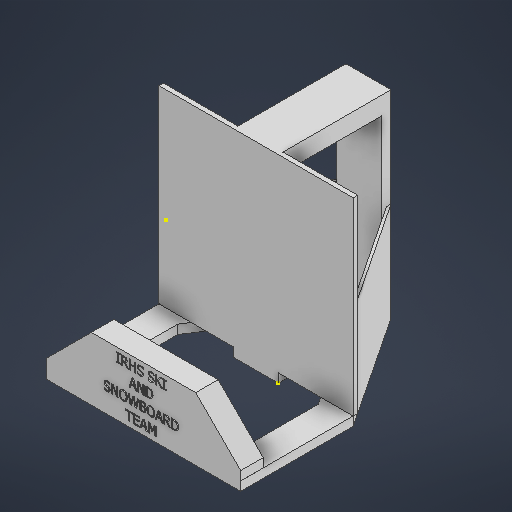
# Autodesk Inventor part: Part2
Saved by Autodesk Inventor 2026 (Build 300175000, 175)
## iProperties
Created: 2025-05-05
Part Number: Part2
Material: Generic
Document SubType Name: Sheet Metal
Designer: 18438
Density: 1 g/cm^3
Sheet Metal Rule: Default_mm
Appearance: Default
Author: 18438
Autodesk Inventor part; units mm, degrees
ref_plane "YZ Plane" through (0, 0, 0) normal (1, 0, 0) x (0, 1, 0)
ref_plane "XZ Plane" through (0, 0, 0) normal (0, 1, 0) x (-1, 0, 0)
ref_plane "XY Plane" through (0, 0, 0) normal (0, 0, 1) x (1, 0, 0)
sketch "Sketch1" plane through (0, 0, 0) normal (0, 1, 0) x (-1, 0, 0)
  line L0 (0, 0) -> (50, 0)
  line L1 (50, 0) -> (50, -250)
  line L2 (50, -250) -> (0, -250)
  line L3 (0, -250) -> (0, 0)
  dimension "d0" = 50
  dimension "d1" = 250
  constraints: 8 end point, 2 parallel, 1 horizontal, 1 perpendicular
  measures "d0" distance of L1.end L2.end
  measures "d1" distance of L0.end L1.end
extrude "Extrusion1" add sketch "Sketch1" along normal blind 20
sketch "Sketch2" plane through (0, 20, 0) normal (0, 1, 0) x (1, 0, 0)
  line L0 (-50, 250) -> (-50, 0) projected
  line L1 (0, 0) -> (0, 250) projected
  line L2 (-50, 0) -> (0, 0)
  line L3 (0, 0) -> (0, 25)
  line L4 (0, 25) -> (-50, 25)
  line L5 (-50, 25) -> (-50, 0)
  point P0 (-50, 25)
  dimension "d4" = 25
  constraints: 8 end point, 2 parallel, 1 horizontal, 1 perpendicular, 1 point on line
  measures "d4" distance of L3.end L2.end
extrude "Extrusion2" add sketch "Sketch2" along normal blind 50
sketch "Sketch3" plane through (0, 20, 0) normal (0, 1, 0) x (1, 0, 0)
  line L0 (0, 25) -> (-50, 25) projected
  line L1 (0, 0) -> (0, 250) projected
  line L2 (-50, 25) -> (0, 25)
  line L3 (0, 25) -> (0, 125)
  line L4 (0, 125) -> (-50, 125)
  line L5 (-50, 125) -> (-50, 25)
  line L6 (-50, 125) -> (0, 125)
  line L7 (0, 125) -> (0, 150)
  line L8 (0, 150) -> (-50, 150)
  line L9 (-50, 150) -> (-50, 125)
  dimension "d7" = 100
  dimension "d8" = 25
  constraints: 16 end point, 4 parallel, 2 horizontal, 2 perpendicular, 1 midpoint, 1 point on line
  measures "d7" distance of L3.end L2.end
  measures "d8" distance of L7.end L6.end
extrude "Extrusion3" add sketch "Sketch3" along normal blind 200 contours L4 L9 L8 L1
sketch "Sketch4" plane through (0, 20, -150) normal (0, 0, -1) x (-1, 0, 0)
  line L0 (0, 0) -> (0, 200) projected
  line L1 (50, 0) -> (50, 200) projected
  line L2 (0, 200) -> (50, 200)
  line L3 (50, 200) -> (50, 170)
  line L4 (50, 170) -> (0, 170)
  line L5 (0, 170) -> (0, 200)
  point P0 (0, -20)
  dimension "d11" = 30
  constraints: 8 end point, 2 parallel, 1 horizontal, 1 perpendicular, 1 point on line
  measures "d11" distance of L2.end L3.end
extrude "Extrusion4" add sketch "Sketch4" along normal blind 100
sketch "Sketch5" plane through (0, 20, 0) normal (0, 1, 0) x (1, 0, 0)
  line L0 (-50, 250) -> (-50, 150) projected
  line L1 (0, 150) -> (0, 250) projected
  line L2 (-50, 250) -> (0, 250)
  line L3 (0, 250) -> (0, 220)
  line L4 (0, 220) -> (-50, 220)
  line L5 (-50, 220) -> (-50, 250)
  point P0 (0, 0)
  dimension "d14" = 30
  constraints: 8 end point, 2 parallel, 1 horizontal, 1 perpendicular, 1 point on line
  measures "d14" distance of L2.end L3.end
extrude "Extrusion5" add sketch "Sketch5" along normal blind 200
sketch "Sketch6" plane through (0, 0, 0) normal (0, -1, 0) x (1, 0, 0)
  line L0 (-50, -125) -> (0, -125) projected
  line L1 (-37.5, -125) -> (-12.5, -125)
  line L2 (-37.5, -125) -> (-12.5, -125)
  line L3 (0, -250) -> (-50, -250) projected
  line L4 (0, -250) -> (82.9156, -125)
  line L5 (-50, -250) -> (-132.9156, -125)
  line L6 (82.9156, -125) -> (57.9156, -108.4169)
  line L7 (57.9156, -108.4169) -> (0, -195.728)
  line L8 (-132.9156, -125) -> (-107.9156, -108.4169)
  line L9 (-107.9156, -108.4169) -> (-50, -195.728)
  line L10 (-50, -220) -> (-50, -150) projected
  line L11 (82.9156, -125) -> (82.9156, 0)
  line L12 (82.9156, 0) -> (52.2372, 0)
  line L13 (52.2372, 0) -> (52.2372, -116.9774)
  line L14 (-132.9156, -125) -> (-132.9156, 0)
  line L15 (-132.9156, -125) -> (-7.9156, -125) construction
  line L16 (-132.9156, 0) -> (-102.9156, 0)
  line L17 (-102.9156, 0) -> (-102.9156, -115.9547)
  line L18 (0, -250) -> (0, -195.728)
  line L19 (0, -150) -> (0, -220) projected
  line L20 (-50, -195.728) -> (-50, -250)
  line L21 (0, -25) -> (-50, -25) projected
  line L22 (0, -25) -> (52.2372, -25)
  line L23 (52.2372, 0) -> (0, 0)
  line L24 (0, 0) -> (-132.9156, 0)
  line L25 (-50, -25) -> (-132.9156, -25)
  point P0 (-25, -125)
  point P1 (-25, -125)
  point P2 (-102.9156, -25)
  dimension "d17" = 25
  dimension "d18" = 25
  dimension "d19" = 150
  dimension "d20" = 150
  dimension "d21" = 30
  dimension "d22" = 30
  dimension "d23" = 90
  dimension "d24" = 30
  constraints: 42 end point, 9 point on line, 6 perpendicular, 4 midpoint, 3 collinear, 3 horizontal, 1 parallel, 1 vertical
  measures "d17" distance of L1.start L1.end
  measures "d18" distance of L2.start L1.end
  measures "d19" distance of L3.start L4.end
  measures "d20" distance of L3.end L5.end
  measures "d21" distance of L4.end L6.end
  measures "d22" distance of L5.end L8.end
  measures "d23" angle of L15 L14
  measures "d24" distance of L14.end L16.end
extrude "Extrusion6" add sketch "Sketch6" against normal blind 10 contours L18 L7 L6 L4 | L5 L8 L9 L10 L20 | L6 L7 L13 L12 L11 | L14 L25 L17 L9 L8 | L14 L16 L17 L25 | L13 L22 L21 L25 L17 L24 L23
sketch "Sketch8" plane through (0, 20, 0) normal (1, 0, 0) x (0, 0, -1)
  line L0 (0, 50) -> (25, 50) projected
  line L1 (0, -20) -> (0, -10) projected
  line L2 (25, 50) -> (0, 50)
  line L3 (0, 50) -> (0, -10)
  line L4 (0, -10) -> (25, -10)
  line L5 (25, -10) -> (25, 50)
  constraints: 8 end point, 2 parallel, 1 horizontal, 1 perpendicular
extrude "Extrusion8" add sketch "Sketch8" along normal blind 83
chamfer "Chamfer1" distance 50 angle 45 1 edges at (83, 70, -12.5)
sketch "Sketch11" plane through (-50, 220, -125) normal (0, 0, 1) x (1, 0, 0)
  point P0 (50, -220)
sketch "Sketch12" plane through (0, 220, 0) normal (0, 1, 0) x (1, 0, 0)
  point P0 (0, 0)
sketch "Sketch13" plane through (0, 20, 0) normal (0, 1, 0) x (1, 0, 0)
  line L0 (0, 125) -> (83, 125) projected
  line L1 (-50, 25) -> (0, 25) projected
  line L2 (0, 125) -> (-50, 125)
  line L3 (-50, 125) -> (-50, 25)
  line L4 (-50, 25) -> (0, 25)
  line L5 (0, 25) -> (0, 125)
  point P0 (0, 0)
  point P1 (0, 25)
  constraints: 8 end point, 2 parallel, 1 horizontal, 1 perpendicular
extrude "Extrusion11" cut sketch "Sketch13" against normal blind 100
sketch "Sketch14" plane through (-50, 0, -125) normal (-1, 0, 0) x (0, 0, 1)
  line L0 (0, 220) -> (-125, 220) projected
  line L1 (9.0453, 10) -> (-70.728, 10) projected
  line L2 (0, 220) -> (-5, 220)
  line L3 (-5, 220) -> (-5, 10)
  line L4 (-5, 10) -> (0, 10)
  line L5 (0, 10) -> (0, 220)
  point P0 (125, 0)
  dimension "d40" = 5
  constraints: 8 end point, 2 parallel, 1 horizontal, 1 perpendicular, 1 point on line
  measures "d40" distance of L4.end L3.end
extrude "Extrusion12" add sketch "Sketch14" along normal blind 83
sketch "Sketch15" plane through (0, 0, -125) normal (1, 0, 0) x (0, 0, -1)
  line L0 (0, 220) -> (125, 220) projected
  line L1 (125, 10) -> (5, 10) projected
  line L2 (0, 220) -> (5, 220)
  line L3 (5, 220) -> (5, 10)
  line L4 (5, 10) -> (0, 10)
  line L5 (0, 10) -> (0, 220)
  point P0 (-125, 0)
  constraints: 8 end point, 2 parallel, 1 horizontal, 1 perpendicular
extrude "Extrusion13" add sketch "Sketch15" along normal blind 83
sketch "Sketch16" plane through (-50, 70, -25) normal (-1, 0, 0) x (0, 0, 1)
  line L0 (0, 0) -> (25, 0) projected
  line L1 (25, -70) -> (25, -60) projected
  line L2 (0, 0) -> (25, 0)
  line L3 (25, 0) -> (25, -60)
  line L4 (25, -60) -> (0, -60)
  line L5 (0, -60) -> (0, 0)
  constraints: 8 end point, 2 parallel, 1 horizontal, 1 perpendicular
extrude "Extrusion14" add sketch "Sketch16" along normal blind 83
chamfer "Chamfer2" distance 50 angle 45 1 edges at (-133, 70, -12.5)
sketch "Sketch17" plane through (0, 10, 0) normal (0, 1, 0) x (1, 0, 0)
  line L0 (-132.9156, 125) -> (-50, 250) projected
  line L1 (-129.599, 130) -> (-50, 250)
  line L2 (-50, 250) -> (-50, 245)
  line L3 (-50, 130) -> (-50, 250) projected
  line L4 (-50, 245) -> (-126.2824, 130)
  line L5 (0, 250) -> (82.9156, 125) projected
  line L6 (79.599, 130) -> (0, 250)
  line L7 (0, 250) -> (0, 245)
  line L8 (0, 130) -> (0, 250) projected
  line L9 (0, 245) -> (76.2824, 130)
  line L10 (0, 130) -> (83, 130) projected
  line L11 (-129.599, 130) -> (-126.2824, 130)
  line L12 (-50, 130) -> (-133, 130) projected
  line L13 (-50, 245) -> (-50, 250)
  point P0 (0, 0)
  dimension "d50" = 5
  dimension "d51" = 5
  constraints: 16 end point, 5 point on line, 3 collinear, 3 parallel
  measures "d50" distance of L0.end L2.end
  measures "d51" distance of L5.start L7.end
extrude "Extrusion15" add sketch "Sketch17" along normal blind 100 contours L0 L2 L4 L11 | L5 L10 L9 L7
sketch "Sketch18" plane through (-50, 190, -220) normal (0, 0, 1) x (1, 0, 0)
  line L0 (0, -170) -> (0, 0) projected
  line L1 (0, 0) -> (50, 0)
  line L2 (50, 0) -> (50, -170)
  line L3 (50, -170) -> (0, -170)
  line L4 (0, -170) -> (0, 0)
  point P0 (50, -190)
  constraints: 8 end point, 2 parallel, 1 horizontal, 1 perpendicular
extrude "Extrusion16" cut sketch "Sketch18" against normal blind 20
sketch "Sketch19" plane through (-50, 190, -150) normal (0, -1, 0) x (1, 0, 0)
  line L0 (50, 0) -> (50, -90) projected
  line L1 (0, 0) -> (50, 0) projected
  line L2 (50, -90) -> (0, -90)
  line L3 (0, -90) -> (0, 0)
  line L4 (0, 0) -> (50, 0)
  line L5 (50, 0) -> (50, -90)
  point P0 (50, 150)
  dimension "d56" = 50
  dimension "d57" = 90
  constraints: 8 end point, 2 parallel, 1 horizontal, 1 perpendicular
  measures "d56" distance of L1.start L4.end
  measures "d57" distance of L2.end L1.start
extrude "Extrusion17" cut sketch "Sketch19" against normal blind 10
sketch "Sketch20" plane through (-132.9156, 0, 0) normal (0, 0, 1) x (1, 0, 0)
  line L0 (72.9869, 65.532) -> (137.8891, 65.532) construction
  line L1 (137.8891, 65.532) -> (137.8891, 62.3556) construction
  line L2 (137.8891, 62.3556) -> (72.9869, 62.3556) construction
  line L3 (72.9869, 62.3556) -> (72.9869, 65.532) construction
  line L4 (81.8127, 55.252) -> (77.9004, 55.252)
  line L5 (77.9004, 55.252) -> (77.9004, 56.2832)
  line L6 (77.9004, 56.2832) -> (79.1854, 56.2832)
  line L7 (79.1854, 56.2832) -> (79.1854, 64.3207)
  line L8 (79.1854, 64.3207) -> (77.9004, 64.3207)
  line L9 (77.9004, 64.3207) -> (77.9004, 65.352)
  line L10 (77.9004, 65.352) -> (81.8127, 65.352)
  line L11 (81.8127, 65.352) -> (81.8127, 64.3207)
  line L12 (81.8127, 64.3207) -> (80.5277, 64.3207)
  line L13 (80.5277, 64.3207) -> (80.5277, 56.2832)
  line L14 (80.5277, 56.2832) -> (81.8127, 56.2832)
  line L15 (81.8127, 56.2832) -> (81.8127, 55.252)
  line L16 (91.2906, 55.252) -> (89.5473, 55.252)
  line L17 (89.5473, 55.252) -> (86.3552, 59.2707)
  line L18 (86.3552, 59.2707) -> (84.8165, 59.2707)
  line L19 (84.8165, 59.2707) -> (84.8165, 55.252)
  line L20 (84.8165, 55.252) -> (83.4742, 55.252)
  line L21 (83.4742, 55.252) -> (83.4742, 65.352)
  line L22 (83.4742, 65.352) -> (86.077, 65.352)
  spline S0 degree 2 poles (86.077, 65.352) (86.9445, 65.352) (88.115, 65.1637) (88.647, 64.82) knots 0 0 0 1 2 2 2
  spline S1 degree 2 poles (88.647, 64.82) (89.179, 64.4762) (89.7928, 63.404) (89.7928, 62.6101) knots 0 0 0 1 2 2 2
  spline S2 degree 2 poles (89.7928, 62.6101) (89.7928, 61.5051) (88.6633, 60.0073) (87.6975, 59.6472) knots 0 0 0 1 2 2 2
  line L23 (87.6975, 59.6472) -> (91.2906, 55.252)
  spline S3 degree 2 poles (88.3932, 62.5037) (88.3932, 62.9456) (88.0822, 63.625) (87.7548, 63.846) knots 0 0 0 1 2 2 2
  spline S4 degree 2 poles (87.7548, 63.846) (87.4684, 64.0342) (86.7072, 64.1897) (86.1506, 64.1897) knots 0 0 0 1 2 2 2
  line L24 (86.1506, 64.1897) -> (84.8165, 64.1897)
  line L25 (84.8165, 64.1897) -> (84.8165, 60.392)
  line L26 (84.8165, 60.392) -> (85.9951, 60.392)
  spline S5 degree 2 poles (85.9951, 60.392) (86.5762, 60.392) (87.5011, 60.5966) (87.8203, 60.9158) knots 0 0 0 1 2 2 2
  spline S6 degree 2 poles (87.8203, 60.9158) (88.115, 61.1941) (88.3932, 61.9798) (88.3932, 62.5037) knots 0 0 0 1 2 2 2
  line L27 (99.4263, 55.252) -> (98.084, 55.252)
  line L28 (98.084, 55.252) -> (98.084, 60.1956)
  line L29 (98.084, 60.1956) -> (93.4351, 60.1956)
  line L30 (93.4351, 60.1956) -> (93.4351, 55.252)
  line L31 (93.4351, 55.252) -> (92.0928, 55.252)
  line L32 (92.0928, 55.252) -> (92.0928, 65.352)
  line L33 (92.0928, 65.352) -> (93.4351, 65.352)
  line L34 (93.4351, 65.352) -> (93.4351, 61.3905)
  line L35 (93.4351, 61.3905) -> (98.084, 61.3905)
  line L36 (98.084, 61.3905) -> (98.084, 65.352)
  line L37 (98.084, 65.352) -> (99.4263, 65.352)
  line L38 (99.4263, 65.352) -> (99.4263, 55.252)
  spline S7 degree 2 poles (104.2881, 55.0719) (103.1913, 55.0719) (101.6526, 55.5302) (100.9732, 55.8576) knots 0 0 0 1 2 2 2
  line L39 (100.9732, 55.8576) -> (100.9732, 57.5437)
  line L40 (100.9732, 57.5437) -> (101.0714, 57.5437)
  spline S8 degree 2 poles (101.0714, 57.5437) (101.7344, 56.9217) (103.4123, 56.2341) (104.1898, 56.2341) knots 0 0 0 1 2 2 2
  spline S9 degree 2 poles (104.1898, 56.2341) (105.303, 56.2341) (106.4406, 57.159) (106.4406, 57.9202) knots 0 0 0 1 2 2 2
  spline S10 degree 2 poles (106.4406, 57.9202) (106.4406, 58.5259) (105.8432, 59.2789) (105.1966, 59.4671) knots 0 0 0 1 2 2 2
  spline S11 degree 2 poles (105.1966, 59.4671) (104.73, 59.5981) (103.9525, 59.7781) (103.3714, 59.9255) knots 0 0 0 1 2 2 2
  spline S12 degree 2 poles (103.3714, 59.9255) (102.8475, 60.0646) (102.0209, 60.482) (101.7017, 60.8176) knots 0 0 0 1 2 2 2
  spline S13 degree 2 poles (101.7017, 60.8176) (101.3906, 61.1532) (101.0469, 62.0535) (101.0469, 62.6428) knots 0 0 0 1 2 2 2
  spline S14 degree 2 poles (101.0469, 62.6428) (101.0469, 63.8705) (102.9621, 65.532) (104.4436, 65.532) knots 0 0 0 1 2 2 2
  spline S15 degree 2 poles (104.4436, 65.532) (105.2948, 65.532) (106.8008, 65.1965) (107.4474, 64.8772) knots 0 0 0 1 2 2 2
  line L41 (107.4474, 64.8772) -> (107.4474, 63.273)
  line L42 (107.4474, 63.273) -> (107.3492, 63.273)
  spline S16 degree 2 poles (107.3492, 63.273) (106.8663, 63.715) (105.3603, 64.3698) (104.5336, 64.3698) knots 0 0 0 1 2 2 2
  spline S17 degree 2 poles (104.5336, 64.3698) (103.6005, 64.3698) (102.4465, 63.494) (102.4465, 62.7819) knots 0 0 0 1 2 2 2
  spline S18 degree 2 poles (102.4465, 62.7819) (102.4465, 62.1435) (103.1258, 61.3823) (103.7642, 61.2105) knots 0 0 0 1 2 2 2
  spline S19 degree 2 poles (103.7642, 61.2105) (104.1898, 61.0959) (105.4257, 60.8012) (105.835, 60.6785) knots 0 0 0 1 2 2 2
  spline S20 degree 2 poles (105.835, 60.6785) (106.8744, 60.3593) (107.8402, 59.0742) (107.8402, 58.133) knots 0 0 0 1 2 2 2
  spline S21 degree 2 poles (107.8402, 58.133) (107.8402, 57.5355) (107.3573, 56.3896) (106.9235, 55.9886) knots 0 0 0 1 2 2 2
  spline S22 degree 2 poles (106.9235, 55.9886) (106.4406, 55.5466) (105.2129, 55.0719) (104.2881, 55.0719) knots 0 0 0 1 2 2 2
  spline S23 degree 2 poles (116.3606, 55.0719) (115.2638, 55.0719) (113.7251, 55.5302) (113.0458, 55.8576) knots 0 0 0 1 2 2 2
  line L43 (113.0458, 55.8576) -> (113.0458, 57.5437)
  line L44 (113.0458, 57.5437) -> (113.144, 57.5437)
  spline S24 degree 2 poles (113.144, 57.5437) (113.8069, 56.9217) (115.4848, 56.2341) (116.2624, 56.2341) knots 0 0 0 1 2 2 2
  spline S25 degree 2 poles (116.2624, 56.2341) (117.3755, 56.2341) (118.5132, 57.159) (118.5132, 57.9202) knots 0 0 0 1 2 2 2
  spline S26 degree 2 poles (118.5132, 57.9202) (118.5132, 58.5259) (117.9157, 59.2789) (117.2691, 59.4671) knots 0 0 0 1 2 2 2
  spline S27 degree 2 poles (117.2691, 59.4671) (116.8026, 59.5981) (116.025, 59.7781) (115.4439, 59.9255) knots 0 0 0 1 2 2 2
  spline S28 degree 2 poles (115.4439, 59.9255) (114.9201, 60.0646) (114.0934, 60.482) (113.7742, 60.8176) knots 0 0 0 1 2 2 2
  spline S29 degree 2 poles (113.7742, 60.8176) (113.4632, 61.1532) (113.1194, 62.0535) (113.1194, 62.6428) knots 0 0 0 1 2 2 2
  spline S30 degree 2 poles (113.1194, 62.6428) (113.1194, 63.8705) (115.0347, 65.532) (116.5161, 65.532) knots 0 0 0 1 2 2 2
  spline S31 degree 2 poles (116.5161, 65.532) (117.3673, 65.532) (118.8733, 65.1965) (119.5199, 64.8772) knots 0 0 0 1 2 2 2
  line L45 (119.5199, 64.8772) -> (119.5199, 63.273)
  line L46 (119.5199, 63.273) -> (119.4217, 63.273)
  spline S32 degree 2 poles (119.4217, 63.273) (118.9388, 63.715) (117.4328, 64.3698) (116.6061, 64.3698) knots 0 0 0 1 2 2 2
  spline S33 degree 2 poles (116.6061, 64.3698) (115.6731, 64.3698) (114.519, 63.494) (114.519, 62.7819) knots 0 0 0 1 2 2 2
  spline S34 degree 2 poles (114.519, 62.7819) (114.519, 62.1435) (115.1983, 61.3823) (115.8368, 61.2105) knots 0 0 0 1 2 2 2
  spline S35 degree 2 poles (115.8368, 61.2105) (116.2624, 61.0959) (117.4983, 60.8012) (117.9075, 60.6785) knots 0 0 0 1 2 2 2
  spline S36 degree 2 poles (117.9075, 60.6785) (118.947, 60.3593) (119.9128, 59.0742) (119.9128, 58.133) knots 0 0 0 1 2 2 2
  spline S37 degree 2 poles (119.9128, 58.133) (119.9128, 57.5355) (119.4299, 56.3896) (118.9961, 55.9886) knots 0 0 0 1 2 2 2
  spline S38 degree 2 poles (118.9961, 55.9886) (118.5132, 55.5466) (117.2855, 55.0719) (116.3606, 55.0719) knots 0 0 0 1 2 2 2
  line L47 (128.6459, 55.252) -> (126.9026, 55.252)
  line L48 (126.9026, 55.252) -> (123.2112, 59.95)
  line L49 (123.2112, 59.95) -> (122.6219, 59.2871)
  line L50 (122.6219, 59.2871) -> (122.6219, 55.252)
  line L51 (122.6219, 55.252) -> (121.2796, 55.252)
  line L52 (121.2796, 55.252) -> (121.2796, 65.352)
  line L53 (121.2796, 65.352) -> (122.6219, 65.352)
  line L54 (122.6219, 65.352) -> (122.6219, 60.7112)
  line L55 (122.6219, 60.7112) -> (126.7634, 65.352)
  line L56 (126.7634, 65.352) -> (128.4004, 65.352)
  line L57 (128.4004, 65.352) -> (124.218, 60.8422)
  line L58 (124.218, 60.8422) -> (128.6459, 55.252)
  line L59 (132.9675, 55.252) -> (129.0552, 55.252)
  line L60 (129.0552, 55.252) -> (129.0552, 56.2832)
  line L61 (129.0552, 56.2832) -> (130.3402, 56.2832)
  line L62 (130.3402, 56.2832) -> (130.3402, 64.3207)
  line L63 (130.3402, 64.3207) -> (129.0552, 64.3207)
  line L64 (129.0552, 64.3207) -> (129.0552, 65.352)
  line L65 (129.0552, 65.352) -> (132.9675, 65.352)
  line L66 (132.9675, 65.352) -> (132.9675, 64.3207)
  line L67 (132.9675, 64.3207) -> (131.6825, 64.3207)
  line L68 (131.6825, 64.3207) -> (131.6825, 56.2832)
  line L69 (131.6825, 56.2832) -> (132.9675, 56.2832)
  line L70 (132.9675, 56.2832) -> (132.9675, 55.252)
  line L71 (91.8595, 38.6226) -> (95.2644, 48.7226)
  line L72 (95.2644, 48.7226) -> (96.9177, 48.7226)
  line L73 (96.9177, 48.7226) -> (100.3225, 38.6226)
  line L74 (100.3225, 38.6226) -> (98.9066, 38.6226)
  line L75 (98.9066, 38.6226) -> (97.9899, 41.4463)
  line L76 (97.9899, 41.4463) -> (94.1349, 41.4463)
  line L77 (94.1349, 41.4463) -> (93.2182, 38.6226)
  line L78 (93.2182, 38.6226) -> (91.8595, 38.6226)
  line L79 (97.6216, 42.5922) -> (96.0583, 47.3475)
  line L80 (96.0583, 47.3475) -> (94.5032, 42.5922)
  line L81 (94.5032, 42.5922) -> (97.6216, 42.5922)
  line L82 (108.5073, 38.6226) -> (107.0013, 38.6226)
  line L83 (107.0013, 38.6226) -> (102.5324, 47.3312)
  line L84 (102.5324, 47.3312) -> (102.5324, 38.6226)
  line L85 (102.5324, 38.6226) -> (101.2802, 38.6226)
  line L86 (101.2802, 38.6226) -> (101.2802, 48.7226)
  line L87 (101.2802, 48.7226) -> (103.1872, 48.7226)
  line L88 (103.1872, 48.7226) -> (107.255, 40.7261)
  line L89 (107.255, 40.7261) -> (107.255, 48.7226)
  line L90 (107.255, 48.7226) -> (108.5073, 48.7226)
  line L91 (108.5073, 48.7226) -> (108.5073, 38.6226)
  spline S39 degree 2 poles (118.5173, 43.6644) (118.5173, 42.2812) (117.396, 40.0549) (116.4547, 39.4329) knots 0 0 0 1 2 2 2
  spline S40 degree 2 poles (116.4547, 39.4329) (115.6853, 38.95) (114.1057, 38.6226) (112.878, 38.6226) knots 0 0 0 1 2 2 2
  line L92 (112.878, 38.6226) -> (110.5535, 38.6226)
  line L93 (110.5535, 38.6226) -> (110.5535, 48.7226)
  line L94 (110.5535, 48.7226) -> (112.8534, 48.7226)
  spline S41 degree 2 poles (112.8534, 48.7226) (114.2776, 48.7226) (115.8981, 48.297) (116.4711, 47.9205) knots 0 0 0 1 2 2 2
  spline S42 degree 2 poles (116.4711, 47.9205) (117.4451, 47.2739) (118.5173, 45.1377) (118.5173, 43.6644) knots 0 0 0 1 2 2 2
  spline S43 degree 2 poles (117.1177, 43.6808) (117.1177, 44.843) (116.3483, 46.4881) (115.5871, 46.9547) knots 0 0 0 1 2 2 2
  spline S44 degree 2 poles (115.5871, 46.9547) (115.0469, 47.2739) (113.8274, 47.5603) (112.9189, 47.5603) knots 0 0 0 1 2 2 2
  line L95 (112.9189, 47.5603) -> (111.8958, 47.5603)
  line L96 (111.8958, 47.5603) -> (111.8958, 39.7848)
  line L97 (111.8958, 39.7848) -> (112.9189, 39.7848)
  spline S45 degree 2 poles (112.9189, 39.7848) (113.811, 39.7848) (115.1615, 40.0713) (115.7099, 40.456) knots 0 0 0 1 2 2 2
  spline S46 degree 2 poles (115.7099, 40.456) (116.4138, 40.9307) (117.1177, 42.5022) (117.1177, 43.6808) knots 0 0 0 1 2 2 2
  spline S47 degree 2 poles (67.4034, 21.8131) (66.3067, 21.8131) (64.7679, 22.2715) (64.0886, 22.5989) knots 0 0 0 1 2 2 2
  line L98 (64.0886, 22.5989) -> (64.0886, 24.2849)
  line L99 (64.0886, 24.2849) -> (64.1868, 24.2849)
  spline S48 degree 2 poles (64.1868, 24.2849) (64.8498, 23.6629) (66.5276, 22.9754) (67.3052, 22.9754) knots 0 0 0 1 2 2 2
  spline S49 degree 2 poles (67.3052, 22.9754) (68.4183, 22.9754) (69.556, 23.9002) (69.556, 24.6614) knots 0 0 0 1 2 2 2
  spline S50 degree 2 poles (69.556, 24.6614) (69.556, 25.2671) (68.9585, 26.0201) (68.3119, 26.2083) knots 0 0 0 1 2 2 2
  spline S51 degree 2 poles (68.3119, 26.2083) (67.8454, 26.3393) (67.0678, 26.5194) (66.4867, 26.6667) knots 0 0 0 1 2 2 2
  spline S52 degree 2 poles (66.4867, 26.6667) (65.9629, 26.8058) (65.1362, 27.2233) (64.817, 27.5588) knots 0 0 0 1 2 2 2
  spline S53 degree 2 poles (64.817, 27.5588) (64.506, 27.8944) (64.1622, 28.7947) (64.1622, 29.384) knots 0 0 0 1 2 2 2
  spline S54 degree 2 poles (64.1622, 29.384) (64.1622, 30.6118) (66.0775, 32.2733) (67.5589, 32.2733) knots 0 0 0 1 2 2 2
  spline S55 degree 2 poles (67.5589, 32.2733) (68.4101, 32.2733) (69.9161, 31.9377) (70.5627, 31.6185) knots 0 0 0 1 2 2 2
  line L100 (70.5627, 31.6185) -> (70.5627, 30.0143)
  line L101 (70.5627, 30.0143) -> (70.4645, 30.0143)
  spline S56 degree 2 poles (70.4645, 30.0143) (69.9816, 30.4562) (68.4756, 31.111) (67.649, 31.111) knots 0 0 0 1 2 2 2
  spline S57 degree 2 poles (67.649, 31.111) (66.7159, 31.111) (65.5618, 30.2353) (65.5618, 29.5232) knots 0 0 0 1 2 2 2
  spline S58 degree 2 poles (65.5618, 29.5232) (65.5618, 28.8848) (66.2412, 28.1236) (66.8796, 27.9517) knots 0 0 0 1 2 2 2
  spline S59 degree 2 poles (66.8796, 27.9517) (67.3052, 27.8371) (68.5411, 27.5425) (68.9503, 27.4197) knots 0 0 0 1 2 2 2
  spline S60 degree 2 poles (68.9503, 27.4197) (69.9898, 27.1005) (70.9556, 25.8155) (70.9556, 24.8742) knots 0 0 0 1 2 2 2
  spline S61 degree 2 poles (70.9556, 24.8742) (70.9556, 24.2767) (70.4727, 23.1309) (70.0389, 22.7298) knots 0 0 0 1 2 2 2
  spline S62 degree 2 poles (70.0389, 22.7298) (69.556, 22.2878) (68.3283, 21.8131) (67.4034, 21.8131) knots 0 0 0 1 2 2 2
  line L102 (79.5496, 21.9932) -> (78.0436, 21.9932)
  line L103 (78.0436, 21.9932) -> (73.5747, 30.7018)
  line L104 (73.5747, 30.7018) -> (73.5747, 21.9932)
  line L105 (73.5747, 21.9932) -> (72.3225, 21.9932)
  line L106 (72.3225, 21.9932) -> (72.3225, 32.0932)
  line L107 (72.3225, 32.0932) -> (74.2295, 32.0932)
  line L108 (74.2295, 32.0932) -> (78.2973, 24.0967)
  line L109 (78.2973, 24.0967) -> (78.2973, 32.0932)
  line L110 (78.2973, 32.0932) -> (79.5496, 32.0932)
  line L111 (79.5496, 32.0932) -> (79.5496, 21.9932)
  spline S63 degree 2 poles (88.7411, 30.9391) (89.314, 30.268) (89.9524, 28.3036) (89.9524, 27.0432) knots 0 0 0 1 2 2 2
  spline S64 degree 2 poles (89.9524, 27.0432) (89.9524, 25.8155) (89.3304, 23.8266) (88.7411, 23.1554) knots 0 0 0 1 2 2 2
  spline S65 degree 2 poles (88.7411, 23.1554) (88.1191, 22.4515) (86.4739, 21.7804) (85.4836, 21.7804) knots 0 0 0 1 2 2 2
  spline S66 degree 2 poles (85.4836, 21.7804) (84.4605, 21.7804) (82.8235, 22.4761) (82.226, 23.1554) knots 0 0 0 1 2 2 2
  spline S67 degree 2 poles (82.226, 23.1554) (81.6449, 23.8266) (81.0229, 25.7991) (81.0229, 27.0432) knots 0 0 0 1 2 2 2
  spline S68 degree 2 poles (81.0229, 27.0432) (81.0229, 28.3118) (81.6531, 30.2434) (82.2342, 30.9391) knots 0 0 0 1 2 2 2
  spline S69 degree 2 poles (82.2342, 30.9391) (82.8235, 31.6103) (84.4686, 32.306) (85.4836, 32.306) knots 0 0 0 1 2 2 2
  spline S70 degree 2 poles (85.4836, 32.306) (86.5148, 32.306) (88.1682, 31.5857) (88.7411, 30.9391) knots 0 0 0 1 2 2 2
  spline S71 degree 2 poles (88.5528, 27.0432) (88.5528, 28.0417) (88.1191, 29.5887) (87.7262, 30.0961) knots 0 0 0 1 2 2 2
  spline S72 degree 2 poles (87.7262, 30.0961) (87.3251, 30.6199) (86.1956, 31.1438) (85.4917, 31.1438) knots 0 0 0 1 2 2 2
  spline S73 degree 2 poles (85.4917, 31.1438) (84.7633, 31.1438) (83.6665, 30.6363) (83.2491, 30.0961) knots 0 0 0 1 2 2 2
  spline S74 degree 2 poles (83.2491, 30.0961) (82.8481, 29.5805) (82.4225, 28.0254) (82.4225, 27.0432) knots 0 0 0 1 2 2 2
  spline S75 degree 2 poles (82.4225, 27.0432) (82.4225, 25.0543) (84.0921, 22.9426) (85.4917, 22.9426) knots 0 0 0 1 2 2 2
  spline S76 degree 2 poles (85.4917, 22.9426) (86.8913, 22.9426) (88.5528, 25.0543) (88.5528, 27.0432) knots 0 0 0 1 2 2 2
  line L112 (102.7452, 32.0932) -> (100.208, 21.9932)
  line L113 (100.208, 21.9932) -> (98.702, 21.9932)
  line L114 (98.702, 21.9932) -> (96.6476, 30.3744)
  line L115 (96.6476, 30.3744) -> (94.6505, 21.9932)
  line L116 (94.6505, 21.9932) -> (93.1609, 21.9932)
  line L117 (93.1609, 21.9932) -> (90.5827, 32.0932)
  line L118 (90.5827, 32.0932) -> (91.9659, 32.0932)
  line L119 (91.9659, 32.0932) -> (93.9957, 23.7202)
  line L120 (93.9957, 23.7202) -> (96.0092, 32.0932)
  line L121 (96.0092, 32.0932) -> (97.376, 32.0932)
  line L122 (97.376, 32.0932) -> (99.4058, 23.622)
  line L123 (99.4058, 23.622) -> (101.4275, 32.0932)
  line L124 (101.4275, 32.0932) -> (102.7452, 32.0932)
  spline S77 degree 2 poles (110.799, 25.0952) (110.799, 24.3422) (110.2261, 23.1882) (109.7514, 22.8117) knots 0 0 0 1 2 2 2
  spline S78 degree 2 poles (109.7514, 22.8117) (109.1785, 22.3697) (107.8771, 21.9932) (106.8458, 21.9932) knots 0 0 0 1 2 2 2
  line L125 (106.8458, 21.9932) -> (103.9484, 21.9932)
  line L126 (103.9484, 21.9932) -> (103.9484, 32.0932)
  line L127 (103.9484, 32.0932) -> (106.6248, 32.0932)
  spline S79 degree 2 poles (106.6248, 32.0932) (107.7052, 32.0932) (108.7856, 31.9541) (109.2767, 31.684) knots 0 0 0 1 2 2 2
  spline S80 degree 2 poles (109.2767, 31.684) (109.825, 31.3975) (110.3243, 30.4562) (110.3243, 29.8178) knots 0 0 0 1 2 2 2
  spline S81 degree 2 poles (110.3243, 29.8178) (110.3243, 29.1058) (109.5713, 27.9763) (108.9084, 27.6571) knots 0 0 0 1 2 2 2
  line L128 (108.9084, 27.6571) -> (108.9084, 27.6079)
  spline S82 degree 2 poles (108.9084, 27.6079) (109.8087, 27.3624) (110.799, 26.061) (110.799, 25.0952) knots 0 0 0 1 2 2 2
  spline S83 degree 2 poles (109.3994, 25.0379) (109.3994, 25.6109) (109.0721, 26.3475) (108.581, 26.6094) knots 0 0 0 1 2 2 2
  spline S84 degree 2 poles (108.581, 26.6094) (108.2618, 26.7731) (107.5088, 26.8713) (106.8131, 26.8713) knots 0 0 0 1 2 2 2
  line L129 (106.8131, 26.8713) -> (105.2907, 26.8713)
  line L130 (105.2907, 26.8713) -> (105.2907, 23.1391)
  line L131 (105.2907, 23.1391) -> (106.3793, 23.1391)
  spline S85 degree 2 poles (106.3793, 23.1391) (107.2632, 23.1391) (108.2781, 23.3028) (108.671, 23.5647) knots 0 0 0 1 2 2 2
  spline S86 degree 2 poles (108.671, 23.5647) (109.0475, 23.8348) (109.3994, 24.5059) (109.3994, 25.0379) knots 0 0 0 1 2 2 2
  spline S87 degree 2 poles (108.9247, 29.6296) (108.9247, 29.9897) (108.6792, 30.5299) (108.4091, 30.6854) knots 0 0 0 1 2 2 2
  spline S88 degree 2 poles (108.4091, 30.6854) (108.0817, 30.8655) (107.2878, 30.9473) (106.5757, 30.9473) knots 0 0 0 1 2 2 2
  line L132 (106.5757, 30.9473) -> (105.2907, 30.9473)
  line L133 (105.2907, 30.9473) -> (105.2907, 27.9926)
  line L134 (105.2907, 27.9926) -> (106.8131, 27.9926)
  spline S89 degree 2 poles (106.8131, 27.9926) (107.4433, 27.9926) (108.0408, 28.1236) (108.36, 28.3282) knots 0 0 0 1 2 2 2
  spline S90 degree 2 poles (108.36, 28.3282) (108.671, 28.5246) (108.9247, 29.1549) (108.9247, 29.6296) knots 0 0 0 1 2 2 2
  spline S91 degree 2 poles (119.2785, 30.9391) (119.8514, 30.268) (120.4898, 28.3036) (120.4898, 27.0432) knots 0 0 0 1 2 2 2
  spline S92 degree 2 poles (120.4898, 27.0432) (120.4898, 25.8155) (119.8678, 23.8266) (119.2785, 23.1554) knots 0 0 0 1 2 2 2
  spline S93 degree 2 poles (119.2785, 23.1554) (118.6564, 22.4515) (117.0113, 21.7804) (116.0209, 21.7804) knots 0 0 0 1 2 2 2
  spline S94 degree 2 poles (116.0209, 21.7804) (114.9978, 21.7804) (113.3609, 22.4761) (112.7634, 23.1554) knots 0 0 0 1 2 2 2
  spline S95 degree 2 poles (112.7634, 23.1554) (112.1823, 23.8266) (111.5602, 25.7991) (111.5602, 27.0432) knots 0 0 0 1 2 2 2
  spline S96 degree 2 poles (111.5602, 27.0432) (111.5602, 28.3118) (112.1904, 30.2434) (112.7716, 30.9391) knots 0 0 0 1 2 2 2
  spline S97 degree 2 poles (112.7716, 30.9391) (113.3609, 31.6103) (115.006, 32.306) (116.0209, 32.306) knots 0 0 0 1 2 2 2
  spline S98 degree 2 poles (116.0209, 32.306) (117.0522, 32.306) (118.7055, 31.5857) (119.2785, 30.9391) knots 0 0 0 1 2 2 2
  spline S99 degree 2 poles (119.0902, 27.0432) (119.0902, 28.0417) (118.6564, 29.5887) (118.2635, 30.0961) knots 0 0 0 1 2 2 2
  spline S100 degree 2 poles (118.2635, 30.0961) (117.8625, 30.6199) (116.733, 31.1438) (116.0291, 31.1438) knots 0 0 0 1 2 2 2
  spline S101 degree 2 poles (116.0291, 31.1438) (115.3007, 31.1438) (114.2039, 30.6363) (113.7865, 30.0961) knots 0 0 0 1 2 2 2
  spline S102 degree 2 poles (113.7865, 30.0961) (113.3854, 29.5805) (112.9598, 28.0254) (112.9598, 27.0432) knots 0 0 0 1 2 2 2
  spline S103 degree 2 poles (112.9598, 27.0432) (112.9598, 25.0543) (114.6295, 22.9426) (116.0291, 22.9426) knots 0 0 0 1 2 2 2
  spline S104 degree 2 poles (116.0291, 22.9426) (117.4287, 22.9426) (119.0902, 25.0543) (119.0902, 27.0432) knots 0 0 0 1 2 2 2
  line L135 (120.8745, 21.9932) -> (124.2793, 32.0932)
  line L136 (124.2793, 32.0932) -> (125.9327, 32.0932)
  line L137 (125.9327, 32.0932) -> (129.3375, 21.9932)
  line L138 (129.3375, 21.9932) -> (127.9216, 21.9932)
  line L139 (127.9216, 21.9932) -> (127.0049, 24.8169)
  line L140 (127.0049, 24.8169) -> (123.1498, 24.8169)
  line L141 (123.1498, 24.8169) -> (122.2332, 21.9932)
  line L142 (122.2332, 21.9932) -> (120.8745, 21.9932)
  line L143 (126.6366, 25.9628) -> (125.0733, 30.7182)
  line L144 (125.0733, 30.7182) -> (123.5182, 25.9628)
  line L145 (123.5182, 25.9628) -> (126.6366, 25.9628)
  line L146 (138.1116, 21.9932) -> (136.3682, 21.9932)
  line L147 (136.3682, 21.9932) -> (133.1762, 26.0119)
  line L148 (133.1762, 26.0119) -> (131.6374, 26.0119)
  line L149 (131.6374, 26.0119) -> (131.6374, 21.9932)
  line L150 (131.6374, 21.9932) -> (130.2951, 21.9932)
  line L151 (130.2951, 21.9932) -> (130.2951, 32.0932)
  line L152 (130.2951, 32.0932) -> (132.8979, 32.0932)
  spline S105 degree 2 poles (132.8979, 32.0932) (133.7655, 32.0932) (134.9359, 31.9049) (135.4679, 31.5612) knots 0 0 0 1 2 2 2
  spline S106 degree 2 poles (135.4679, 31.5612) (135.9999, 31.2174) (136.6138, 30.1452) (136.6138, 29.3513) knots 0 0 0 1 2 2 2
  spline S107 degree 2 poles (136.6138, 29.3513) (136.6138, 28.2464) (135.4843, 26.7485) (134.5185, 26.3884) knots 0 0 0 1 2 2 2
  line L153 (134.5185, 26.3884) -> (138.1116, 21.9932)
  spline S108 degree 2 poles (135.2142, 29.2449) (135.2142, 29.6869) (134.9032, 30.3662) (134.5758, 30.5872) knots 0 0 0 1 2 2 2
  spline S109 degree 2 poles (134.5758, 30.5872) (134.2893, 30.7754) (133.5281, 30.931) (132.9716, 30.931) knots 0 0 0 1 2 2 2
  line L154 (132.9716, 30.931) -> (131.6374, 30.931)
  line L155 (131.6374, 30.931) -> (131.6374, 27.1332)
  line L156 (131.6374, 27.1332) -> (132.8161, 27.1332)
  spline S110 degree 2 poles (132.8161, 27.1332) (133.3972, 27.1332) (134.3221, 27.3378) (134.6413, 27.6571) knots 0 0 0 1 2 2 2
  spline S111 degree 2 poles (134.6413, 27.6571) (134.9359, 27.9353) (135.2142, 28.7211) (135.2142, 29.2449) knots 0 0 0 1 2 2 2
  spline S112 degree 2 poles (146.8775, 27.035) (146.8775, 25.6518) (145.7562, 23.4255) (144.8149, 22.8035) knots 0 0 0 1 2 2 2
  spline S113 degree 2 poles (144.8149, 22.8035) (144.0456, 22.3206) (142.4659, 21.9932) (141.2382, 21.9932) knots 0 0 0 1 2 2 2
  line L157 (141.2382, 21.9932) -> (138.9137, 21.9932)
  line L158 (138.9137, 21.9932) -> (138.9137, 32.0932)
  line L159 (138.9137, 32.0932) -> (141.2136, 32.0932)
  spline S114 degree 2 poles (141.2136, 32.0932) (142.6378, 32.0932) (144.2584, 31.6676) (144.8313, 31.2911) knots 0 0 0 1 2 2 2
  spline S115 degree 2 poles (144.8313, 31.2911) (145.8053, 30.6445) (146.8775, 28.5083) (146.8775, 27.035) knots 0 0 0 1 2 2 2
  spline S116 degree 2 poles (145.4779, 27.0514) (145.4779, 28.2136) (144.7085, 29.8588) (143.9473, 30.3253) knots 0 0 0 1 2 2 2
  spline S117 degree 2 poles (143.9473, 30.3253) (143.4071, 30.6445) (142.1876, 30.931) (141.2791, 30.931) knots 0 0 0 1 2 2 2
  line L160 (141.2791, 30.931) -> (140.256, 30.931)
  line L161 (140.256, 30.931) -> (140.256, 23.1554)
  line L162 (140.256, 23.1554) -> (141.2791, 23.1554)
  spline S118 degree 2 poles (141.2791, 23.1554) (142.1712, 23.1554) (143.5217, 23.4419) (144.0701, 23.8266) knots 0 0 0 1 2 2 2
  spline S119 degree 2 poles (144.0701, 23.8266) (144.774, 24.3013) (145.4779, 25.8728) (145.4779, 27.0514) knots 0 0 0 1 2 2 2
  line L163 (91.3479, 5.3638) -> (91.3479, 14.2688)
  line L164 (91.3479, 14.2688) -> (87.9594, 14.2688)
  line L165 (87.9594, 14.2688) -> (87.9594, 15.4638)
  line L166 (87.9594, 15.4638) -> (96.0787, 15.4638)
  line L167 (96.0787, 15.4638) -> (96.0787, 14.2688)
  line L168 (96.0787, 14.2688) -> (92.6902, 14.2688)
  line L169 (92.6902, 14.2688) -> (92.6902, 5.3638)
  line L170 (92.6902, 5.3638) -> (91.3479, 5.3638)
  line L171 (97.1018, 5.3638) -> (97.1018, 15.4638)
  line L172 (97.1018, 15.4638) -> (103.4205, 15.4638)
  line L173 (103.4205, 15.4638) -> (103.4205, 14.2688)
  line L174 (103.4205, 14.2688) -> (98.4441, 14.2688)
  line L175 (98.4441, 14.2688) -> (98.4441, 11.5024)
  line L176 (98.4441, 11.5024) -> (103.0849, 11.5024)
  line L177 (103.0849, 11.5024) -> (103.0849, 10.3074)
  line L178 (103.0849, 10.3074) -> (98.4441, 10.3074)
  line L179 (98.4441, 10.3074) -> (98.4441, 6.5588)
  line L180 (98.4441, 6.5588) -> (103.4205, 6.5588)
  line L181 (103.4205, 6.5588) -> (103.4205, 5.3638)
  line L182 (103.4205, 5.3638) -> (97.1018, 5.3638)
  line L183 (103.8052, 5.3638) -> (107.21, 15.4638)
  line L184 (107.21, 15.4638) -> (108.8633, 15.4638)
  line L185 (108.8633, 15.4638) -> (112.2682, 5.3638)
  line L186 (112.2682, 5.3638) -> (110.8522, 5.3638)
  line L187 (110.8522, 5.3638) -> (109.9355, 8.1876)
  line L188 (109.9355, 8.1876) -> (106.0805, 8.1876)
  line L189 (106.0805, 8.1876) -> (105.1638, 5.3638)
  line L190 (105.1638, 5.3638) -> (103.8052, 5.3638)
  line L191 (109.5672, 9.3334) -> (108.0039, 14.0888)
  line L192 (108.0039, 14.0888) -> (106.4488, 9.3334)
  line L193 (106.4488, 9.3334) -> (109.5672, 9.3334)
  line L194 (121.8853, 5.3638) -> (120.543, 5.3638)
  line L195 (120.543, 5.3638) -> (120.543, 14.0642)
  line L196 (120.543, 14.0642) -> (117.9075, 8.1466)
  line L197 (117.9075, 8.1466) -> (117.089, 8.1466)
  line L198 (117.089, 8.1466) -> (114.4781, 14.0642)
  line L199 (114.4781, 14.0642) -> (114.4781, 5.3638)
  line L200 (114.4781, 5.3638) -> (113.2258, 5.3638)
  line L201 (113.2258, 5.3638) -> (113.2258, 15.4638)
  line L202 (113.2258, 15.4638) -> (115.0592, 15.4638)
  line L203 (115.0592, 15.4638) -> (117.5801, 9.8409)
  line L204 (117.5801, 9.8409) -> (120.0192, 15.4638)
  line L205 (120.0192, 15.4638) -> (121.8853, 15.4638)
  line L206 (121.8853, 15.4638) -> (121.8853, 5.3638)
  point P0 (132.9156, 0)
  dimension "MinimumRemnant" = 1
  constraints: 2 other
extrude "Extrusion18" cut sketch "Sketch20" against normal blind 1
equation "\"MinimumRemnant\" = 2 * Thickness"
equation "\"BendRadius\" = Thickness"
equation "\"BendReliefWidth\" = Thickness"
equation "\"BendReliefDepth\" = 0.5 * Thickness"
equation "\"CornerReliefSize\" = 4 * Thickness"
equation "\"TransitionRadius\" = BendRadius"
equation "\"JacobiRadiusSize\" = BendRadius"
equation "\"GapSize\" = Thickness"
equation "\"Thickness\" = 0.5"
body "Solid1"
